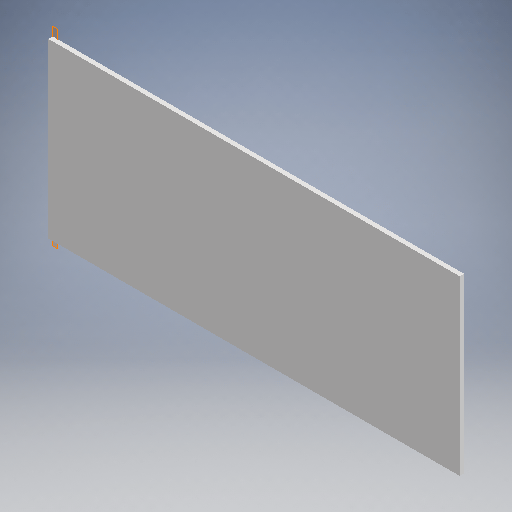
# Autodesk Inventor part: RIGHT WALL
Saved by Autodesk Inventor 2025.2 (Build 292293000, 293)
## iProperties
Created: 2025-01-27
Part Number: RIGHT WALL
Material: Generic
Document SubType Name: Modeling
Designer: Anna
Density: 1 g/cm^3
Appearance: Default
Author: Anna
Autodesk Inventor part; units mm, degrees
ref_plane "YZ Plane" through (0, 0, 0) normal (1, 0, 0) x (0, 1, 0)
ref_plane "XZ Plane" through (0, 0, 0) normal (0, 1, 0) x (-1, 0, 0)
ref_plane "XY Plane" through (0, 0, 0) normal (0, 0, 1) x (1, 0, 0)
ref_plane "Work Plane2" through (0, 0, 0) normal (0, 0, 1) x (1, 0, 0)
sketch "Sketch2" plane through (0, 0, 0) normal (0, 0, 1) x (1, 0, 0)
  line L0 (0, 0) -> (0, -1003.3) projected
  line L1 (0, -1003.3) -> (2387.6, -1003.3)
  line L2 (2387.6, -1003.3) -> (2387.6, 0)
  line L3 (2387.6, 0) -> (0, 0)
  dimension "d0" = 2387.6
  constraints: 6 end point, 1 horizontal, 1 perpendicular, 1 vertical
  measures "d0" distance of L0.end L1.end
extrude "Extrusion1" add sketch "Sketch2" along normal blind 25.4
body "Solid1"
